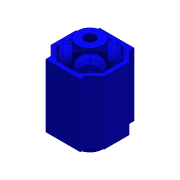
# Autodesk Inventor part: Quad
Saved by Autodesk Inventor 2022.2 (Build 262287010, 287A)
## iProperties
RuleStatus: InUse
Created: 2021-06-15
Part Number: Quad
Material: Generic
Document SubType Name: Modeling
Designer: Josep
Density: 1 g/cm^3
Appearance: Quadrupole
Mass: 2915.59 g
Surface Area: 5027.97 cm^2
Volume: 2915.59 cm^3
Author: Josep
Autodesk Inventor part; units mm, degrees
ref_plane "YZ Plane" through (0, 0, 0) normal (1, 0, 0) x (0, 1, 0)
ref_plane "XZ Plane" through (0, 0, 0) normal (0, 1, 0) x (-1, 0, 0)
ref_plane "XY Plane" through (0, 0, 0) normal (0, 0, 1) x (1, 0, 0)
sketch "Sketch1" plane through (0, 0, 0) normal (0, 0, 1) x (0, 1, 0)
  line L0 (75, 0) -> (63, 0)
  line L1 (75, 0) -> (75, -33.9289)
  line L2 (59.4645, -49.4645) -> (33.9289, -75)
  line L3 (33.9289, -75) -> (0, -75)
  line L4 (0, -75) -> (0, -63)
  line L5 (0, -63) -> (28.9584, -63)
  line L6 (28.9584, -63) -> (63, -28.9584)
  line L7 (63, -28.9584) -> (63, 0)
  line L8 (58.594, -33.3644) -> (30.2714, -5.0419)
  line L9 (33.3644, -58.594) -> (5.0419, -30.2714)
  arc A0 (30.2714, -5.0419) -> (5.0419, -30.2714) centre (29.0086, -29.0086) ccw
  line L10 (58.594, -33.3644) -> (33.3644, -58.594)
  line L11 (75, -33.9289) -> (75, -48)
  line L12 (75, -48) -> (63, -48)
  arc A1 (63, -48) -> (59.4645, -49.4645) centre (63, -53) ccw
  line L13 (10.242, -35.4716) -> (15.0786, -30.635)
  line L14 (15.0786, -30.635) -> (38.201, -53.7574)
  line L15 (35.4716, -10.242) -> (30.635, -15.0786)
  line L16 (30.635, -15.0786) -> (53.7574, -38.201)
  line L17 (90.1153, 0) -> (-15.6921, 0) projected
  line L18 (0, 15.6921) -> (0, -90.1153) projected
  point P0 (0, 0)
  point P1 (45.9792, -45.9792)
  point P2 (38.201, -53.7574)
  point P3 (53.7574, -38.201)
  dimension "d9" = 12
  dimension "d10" = 12
  dimension "d13" = 35.68
  dimension "d15" = 24
  dimension "d41" = 24
  dimension "d44" = 5
  dimension "d45" = 12
  dimension "d46" = 135
  dimension "d47" = 6.84
  dimension "d49" = 32.7
  dimension "d80" = 75
  dimension "d81" = 48
  constraints: 34 end point, 6 point on line, 5 equal length, 4 collinear, 4 point on circle, 3 horizontal, 3 parallel, 3 perpendicular, 2 centre point, 2 midpoint, 2 tangent, 2 vertical
  measures "d9" distance between parallel lines of L6 L2
  measures "d10" distance between parallel lines of L7 L1
  measures "d13" distance between parallel lines of L9 L8
  measures "d15" radius of A0
  measures "d41" distance from line of L6 A0.centre
  measures "d44" radius of A1
  measures "d45" distance of L11.end L12.end
  measures "d46" angle of L7 L6
  measures "d47" distance of L13.start L13.end
  measures "d49" distance of L13.end L14.end
  measures "d80" distance between parallel lines of L18 L1
  measures "d81" distance between parallel lines of L12 L17
extrude "Extrusion1" add sketch "Sketch1" along normal mid plane 175 contours L1 L11 L12 A1 L2 L3 L4 L5 L6 L7 L0 | L6 L14 L13 L9 A0 L8 L15 L16
sketch "Sketch6" plane through (63, 28.9584, -87.5) normal (-0.7071068, -0.7071068, 0) x (0, 0, 1)
  line L0 (0, -16.9706) -> (0, 0) projected
  line L1 (0, 0) -> (0, 13.0711) projected
  line L2 (0, 13.0711) -> (0, 35.0711) projected
  line L3 (0, 35.0711) -> (0, 48.1421) projected
  line L4 (0, 48.1421) -> (0, 65.1127) projected
  line L5 (0, 65.1127) -> (175, 65.1127) projected
  line L6 (175, 65.1127) -> (175, 48.1421) projected
  line L7 (175, 48.1421) -> (175, 35.0711) projected
  line L8 (175, 35.0711) -> (175, 13.0711) projected
  line L9 (175, 13.0711) -> (175, 0) projected
  line L10 (175, 0) -> (175, -16.9706) projected
  line L11 (175, -16.9706) -> (0, -16.9706) projected
  line L12 (0, 0) -> (175, 0) projected
  line L13 (175, 13.0711) -> (0, 13.0711) projected
  line L14 (0, 35.0711) -> (175, 35.0711) projected
  line L15 (175, 48.1421) -> (0, 48.1421) projected
  line L16 (166, 35.0711) -> (175, 26.0711)
  line L17 (175, 26.0711) -> (175, 22.0711)
  line L18 (175, 22.0711) -> (166, 13.0711)
  point P0 (87.5, 24.0711)
  point P1 (175, 24.0711)
  point P2 (175, 24.0711)
  dimension "d50" = 0
  dimension "d51" = 4
  dimension "d52" = 9
  constraints: 6 end point, 2 midpoint, 2 point on line, 1 coincident, 1 collinear, 1 vertical alignment
  measures "d50" distance between parallel lines of L17 L8
  measures "d51" distance of L16.end L17.end
  measures "d52" distance from line of L18.end L17
extrude "Extrusion4" cut sketch "Sketch6" along normal up to surface (32.7 mm away) contours L18 L8 L13 | L14 L8 L16
sketch "Sketch7" plane through (0, 0, 87.5) normal (0, 0, 1) x (1, 0, 0)
  line L0 (21.4426, 24.271) -> (10.242, 35.4716) projected
  line L1 (10.242, 35.4716) -> (5.0419, 30.2714) projected
  arc A0 (5.0419, 30.2714) -> (30.2714, 5.0419) centre (29.0086, 29.0086) ccw projected
  line L2 (30.2714, 5.0419) -> (35.4716, 10.242) projected
  line L3 (35.4716, 10.242) -> (24.271, 21.4426) projected
  line L4 (24.271, 21.4426) -> (47.3934, 44.565) projected
  line L5 (47.3934, 44.565) -> (63, 28.9584) projected
  line L6 (63, 28.9584) -> (63, 0) projected
  line L7 (63, 0) -> (75, 0) projected
  line L8 (75, 0) -> (75, 33.9289) projected
  line L9 (75, 33.9289) -> (49.4645, 59.4645) projected
  arc A1 (48, 63) -> (49.4645, 59.4645) centre (53, 63) ccw projected
  line L10 (48, 63) -> (48, 75) projected
  line L11 (48, 75) -> (0, 75) projected
  line L12 (0, 75) -> (0, 63) projected
  line L13 (0, 63) -> (28.9584, 63) projected
  line L14 (28.9584, 63) -> (44.565, 47.3934) projected
  line L15 (44.565, 47.3934) -> (21.4426, 24.271) projected
  line L16 (21.4426, 24.271) -> (24.271, 21.4426)
  point P0 (0, 0)
  constraints: 2 end point
extrude "Extrusion5" add sketch "Sketch7" along normal blind 15.3 contours L16 L3 L2 A0 L1 L0
sketch "Sketch8" plane through (0, 0, 0) normal (0, 0, 1) x (0, 1, 0)
  line L0 (10.242, -35.4716) -> (5.0419, -30.2714) projected
  arc A0 (30.2714, -5.0419) -> (5.0419, -30.2714) centre (29.0086, -29.0086) ccw projected
  line L1 (30.2714, -5.0419) -> (35.4716, -10.242) projected
  line L2 (35.4716, -10.242) -> (30.635, -15.0786) projected
  line L3 (30.635, -15.0786) -> (53.7574, -38.201) projected
  line L4 (53.7574, -38.201) -> (63, -28.9584) projected
  line L5 (63, -28.9584) -> (63, 0) projected
  line L6 (75, -48) -> (63, -48) projected
  arc A1 (63, -48) -> (59.4645, -49.4645) centre (63, -53) ccw projected
  line L7 (59.4645, -49.4645) -> (33.9289, -75) projected
  line L8 (33.9289, -75) -> (0, -75) projected
  line L9 (0, -75) -> (0, -63) projected
  line L10 (0, -63) -> (28.9584, -63) projected
  line L11 (28.9584, -63) -> (38.201, -53.7574) projected
  line L12 (38.201, -53.7574) -> (15.0786, -30.635) projected
  line L13 (15.0786, -30.635) -> (10.242, -35.4716) projected
  line L14 (60.7931, -25.5084) -> (52.3431, -33.9584)
  line L15 (52.3431, -33.9584) -> (33.6755, -15.2908)
  line L16 (33.6755, -15.2908) -> (48.0298, -0.9365)
  line L17 (48.0298, -0.9365) -> (60.7931, -13.6998)
  line L18 (60.7931, -13.6998) -> (60.7931, -25.5084)
  line L19 (63, 0) -> (75, 0) projected
  line L20 (75, 0) -> (75, -48) projected
  dimension "d83" = 13
  dimension "d84" = 20.3
  dimension "d85" = 18.05
  dimension "d86" = 4
  dimension "d87" = 26.4
  constraints: 10 end point, 4 parallel, 1 perpendicular
  measures "d83" distance from line of A0.centre L15
  measures "d84" distance of L15.end L16.end
  measures "d85" distance of L16.end L17.end
  measures "d86" distance between parallel lines of L4 L14
  measures "d87" distance of L14.end L15.end
sketch "Sketch9" plane through (10.242, 35.4716, 102.8) normal (0.7071068, 0.7071068, 0) x (0, 0, -1)
  line L0 (24, 5.31) -> (181.6, 5.31)
  line L1 (204.6, -17.69) -> (204.6, -17.99)
  line L2 (181.6, -40.99) -> (24, -40.99)
  line L3 (1, -17.99) -> (1, -17.69)
  line L4 (0, -35.68) -> (0, 0) projected
  arc A0 (1, -17.99) -> (24, -40.99) centre (24, -17.99) ccw
  arc A1 (24, 5.31) -> (1, -17.69) centre (24, -17.69) ccw
  arc A2 (181.6, -40.99) -> (204.6, -17.99) centre (181.6, -17.99) ccw
  arc A3 (204.6, -17.69) -> (181.6, 5.31) centre (181.6, -17.69) ccw
  point P0 (102.8, -17.84)
  point P1 (102.8, 5.31)
  point P2 (1, -17.84)
  point P3 (0, -17.84)
  point P4 (102.8, -40.99)
  dimension "d64" = 23
  dimension "d65" = 23
  dimension "d68" = 1
  constraints: 8 end point, 8 point on circle, 8 tangent, 4 centre point, 4 midpoint, 2 equal radius, 2 parallel, 1 horizontal, 1 horizontal alignment, 1 perpendicular, 1 vertical alignment
  measures "d64" radius of A0
  measures "d65" radius of A2
  measures "d68" distance of point (1, -17.84) point (0, -17.84)
sweep "Sweep2" add profiles "Sketch8" path "Sketch9" path curves L0 A3 L1 A2 L2 A0 L3 A1 contours L14 L15 L16 L17 L18
mirror "Mirror5" about plane through (0, 0, 0) normal (1, 0, 0)
mirror "Mirror3" about plane through (0, 0, 0) normal (0, 1, 0)
sketch "Sketch4" plane through (0, 0, 0) normal (0, 0, 1) x (0, 1, 0)
  circle A0 centre (0, 0) radius 15.875
  circle A1 centre (0, 0) radius 15.113
  dimension "d69" = 31.75
  dimension "d70" = 30.226
  constraints: 2 centre point, 2 coincident
  measures "d69" diameter of A0
  measures "d70" diameter of A1
extrude "Extrusion2" add sketch "Sketch4" along normal mid plane 250
sketch "Sketch5" plane through (0, 0, 125) normal (0, 0, 1) x (1, 0, 0)
  circle A0 centre (0, 0) radius 34.925
  circle A1 centre (0, 0) radius 15.113 projected
  point P0 (5.0095, 29.2154)
  point P1 (0, 15.113)
  dimension "d71" = 69.85
  constraints: 1 centre point, 1 coincident, 1 other
  measures "d71" diameter of A0
extrude "Extrusion3" add sketch "Sketch5" against normal blind 12.7
mirror "Mirror1" about plane through (0, 0, 0) normal (0, 0, 1) of "Extrusion3"
body "Solid1"
